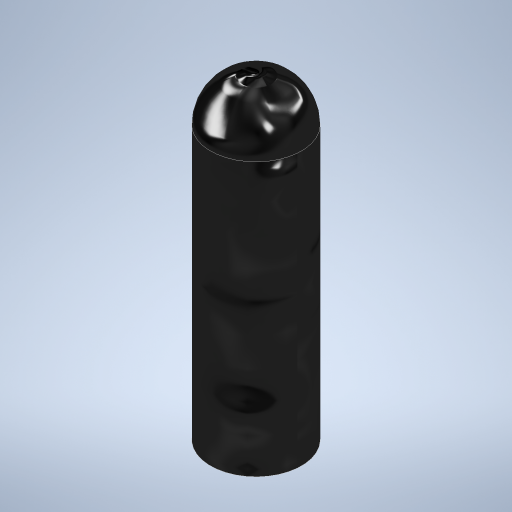
# Autodesk Inventor part: Stift_kurz
Saved by Autodesk Inventor 2024 (Build 280153000, 153)
## iProperties
Created: 2023-08-23
Part Number: Stift_kurz
Material: Generisch
Document SubType Name: Modeling
Designer: rapp
Density: 1 g/cm^3
Appearance: Schwarz
Author: rapp
Autodesk Inventor part; units mm, degrees
ref_plane "YZ Plane" through (0, 0, 0) normal (1, 0, 0) x (0, 1, 0)
ref_plane "XZ Plane" through (0, 0, 0) normal (0, 1, 0) x (-1, 0, 0)
ref_plane "XY Plane" through (0, 0, 0) normal (0, 0, 1) x (1, 0, 0)
sketch "Skizze1" plane through (0, 0, 0) normal (0, 1, 0) x (-1, 0, 0)
  arc A0 (5, -5) -> (0, 0) centre (0, -5) ccw
  line L0 (7.2426, 0) -> (-1.2071, 0) projected
  line L1 (0, -42.2071) -> (0, 8.2426) projected
  line L2 (5, -35) -> (5, -5)
  line L3 (0, 0) -> (0, -35)
  line L4 (0, 0) -> (0, -35)
  line L5 (5, -35) -> (0, -35)
  dimension "d0" = 10
  dimension "d2" = 30
  constraints: 8 end point, 2 point on circle, 2 tangent, 1 centre point, 1 perpendicular
  measures "d0" diameter of A0
  measures "d2" distance of L2.end L2.start
revolve "Umdrehung1" add sketch "Skizze1" angle 360 about axis through (0, 0, -10) along (0, 0, 1)
